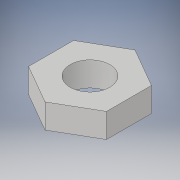
# Autodesk Inventor part: Crossbeam to LS Nut
Saved by Autodesk Inventor 2017 (Build 210142000, 142)
## iProperties
Created: 2016-09-26
Part Number: Crossbeam to LS Nut
Material: Generic
Document SubType Name: Modeling
Designer: Hanson
Density: 1 g/cm^3
Appearance: Default
Author: Hanson
Autodesk Inventor part; units mm, degrees
ref_plane "YZ Plane" through (0, 0, 0) normal (1, 0, 0) x (0, 1, 0)
ref_plane "XZ Plane" through (0, 0, 0) normal (0, 1, 0) x (-1, 0, 0)
ref_plane "XY Plane" through (0, 0, 0) normal (0, 0, 1) x (1, 0, 0)
sketch "Sketch3" plane through (0, 0, 0) normal (0, 1, 0) x (-1, 0, 0)
  line L0 (0, -5.8659) -> (-5.08, -2.9329)
  line L1 (-5.08, -2.9329) -> (-5.08, 2.9329)
  line L2 (-5.08, 2.9329) -> (0, 5.8659)
  line L3 (0, 5.8659) -> (5.08, 2.9329)
  line L4 (5.08, 2.9329) -> (5.08, -2.9329)
  line L5 (5.08, -2.9329) -> (0, -5.8659)
  point P0 (0, 0)
  point P1 (0, 0)
  dimension "d10" = 5.08
  constraints: 12 end point, 1 coincident, 13 other
  measures "d10" distance from line of L3 point (0, 0)
extrude "Extrusion2" add sketch "Sketch3" along normal blind 3.175
sketch "Sketch4" plane through (0, 3.175, 0) normal (0, 1, 0) x (1, 0, 0)
  point P0 (0, 0)
  point P1 (0, 0)
  constraints: 1 coincident
hole "Hole2" at (0, 3.175, 0) direction (0, -1, 0) diameter 5.1562 end through all
body "Solid2"
